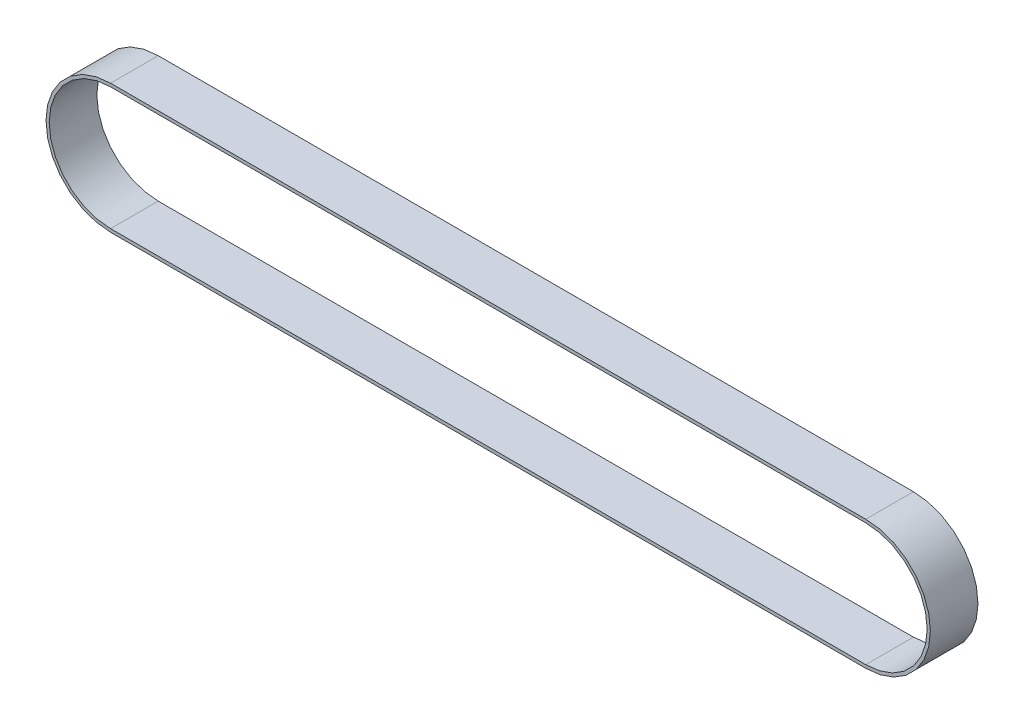
# Autodesk Inventor part: Belt
Saved by Autodesk Inventor 2025.2 (Build 292293000, 293)
## iProperties
Created: 2024-11-14
Part Number: Belt
Material: Generic
Document SubType Name: Modeling
Designer: JL
Density: 1 g/cm^3
Appearance: Default
Author: JL
Autodesk Inventor part; units mm, degrees
sketch "Sketch1" plane through (0, 0, 0) normal (0, 0, 1) x (1, 0, 0)
  circle A0 centre (0, 0) radius 19.3229 construction
  arc A1 (0, 19.8229) -> (0, -19.8229) centre (0, 0) ccw construction
  line L0 (0, 19.8229) -> (237.7246, 19.8229) construction
  line L1 (0, -19.8229) -> (237.7246, -19.8229) construction
  arc A2 (237.7246, -19.8229) -> (237.7246, 19.8229) centre (237.7246, 0) ccw construction
  line L2 (237.7246, 19.3229) -> (0, 19.3229)
  arc A3 (0, 19.3229) -> (0, -19.3229) centre (0, 0) ccw
  line L3 (0, -19.3229) -> (237.7246, -19.3229)
  arc A4 (237.7246, -19.3229) -> (237.7246, 19.3229) centre (237.7246, 0) ccw
  line L4 (237.7246, 20.3229) -> (0, 20.3229)
  arc A5 (0, 20.3229) -> (0, -20.3229) centre (0, 0) ccw
  line L5 (0, -20.3229) -> (237.7246, -20.3229)
  arc A6 (237.7246, -20.3229) -> (237.7246, 20.3229) centre (237.7246, 0) ccw
  point P0 (0, 0)
  dimension "pitch_line_distance" = 0.5
  dimension "end_arc_length" = 62.2754
  dimension "d5" = 237.7246
  dimension "d6" = 0.5
  dimension "d7" = 0.5
  constraints: 12 end point, 12 point on circle, 6 centre point, 4 tangent, 2 horizontal, 6 other
  measures "pitch_line_distance" radial gap between concentric circles of A0 A1
  measures "d5" distance of L0.start L0.end
  measures "d6" distance between parallel lines of L0 L2
  measures "d7" distance between parallel lines of L0 L4
ref_plane "Work Plane1" through (-31.1735, -31.1443, -7.5) normal (0, 0, -1) x (-0.3091, 0.951, 0)
ref_plane "Work Plane2" through (-25.9469, -25.926, 7.5) normal (0, 0, 1) x (0.9988, -0.0499, 0)
ref_plane "Work Plane3" through (-31.1735, -31.1443, -7.5) normal (0, 0, -1) x (-0.3091, 0.951, 0)
extrude "Extrusion2" add sketch "Sketch1" against normal up to surface (15 mm away) from surface at 7.5
equation "\"d5\" = 0.5 * length - end_arc_length"
equation "\"d6\" = pitch_line_distance"
equation "\"d7\" = pitch_line_distance"
equation "\"length\" = 600"
body "Solid2"
